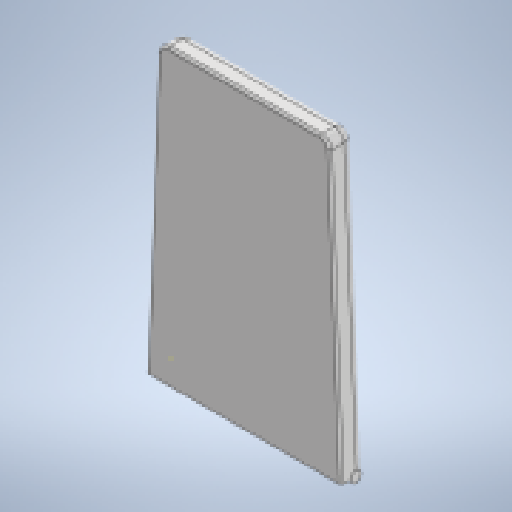
# Autodesk Inventor part: backrest wheelchair EG26
Saved by Autodesk Inventor 2023 (Build 270158000, 158)
## iProperties
Created: 2023-10-18
Part Number: backrest wheelchair EG26
Material: Generic
Document SubType Name: Modeling
Designer: user
Density: 1 g/cm^3
Appearance: Default
Author: user
Autodesk Inventor part; units mm, degrees
ref_plane "YZ Plane" through (0, 0, 0) normal (1, 0, 0) x (0, 1, 0)
ref_plane "XZ Plane" through (0, 0, 0) normal (0, 1, 0) x (-1, 0, 0)
ref_plane "XY Plane" through (0, 0, 0) normal (0, 0, 1) x (1, 0, 0)
sketch "Sketch1" plane through (0, 0, 0) normal (0, 0, 1) x (1, 0, 0)
  line L0 (0, 0) -> (25, 600)
  line L1 (25, 600) -> (375, 600)
  line L2 (375, 600) -> (400, 0)
  line L3 (400, 0) -> (0, 0)
  arc A0 (120.3096, 600) -> (279.6904, 600) centre (200, 673.1568) ccw
  line L4 (120.3096, 600) -> (25, 600)
  line L5 (25, 600) -> (0, 0)
  dimension "d0" = 600
  dimension "d1" = 25
  dimension "d2" = 350
  dimension "d3" = 400
  dimension "d4" = 175
  constraints: 12 end point, 2 point on circle, 2 point on line, 1 centre point, 1 collinear, 1 horizontal, 1 parallel
  measures "d0" vertical distance of L0.start L0.end
  measures "d1" horizontal distance of L0.start L0.end
  measures "d2" distance of L0.end L1.end
  measures "d3" distance of L2.end L0.start
  measures "d4" horizontal distance of L1.end A0.centre
extrude "Extrusion1" add sketch "Sketch1" along normal blind 50
fillet "Fillet1" radius 20 5 edges at (200, 600, 0) (387.5, 300, 0) (12.5, 300, 0) (25, 600, 25) (375, 600, 25)
fillet "Fillet2" radius 5 5 edges at (200, 600, 50) (30.3394, 594.4335, 50) (369.6606, 594.4335, 50) (387.8993, 290.4163, 50) (12.1007, 290.4163, 50)
sketch "Sketch2" plane through (0, 0, 0) normal (0, 0, 1) x (1, 0, 0)
  point P0 (0, 0)
sketch "Sketch3" plane through (0, 0, 0) normal (1, 0, 0) x (0, 1, 0)
  line L0 (0, 0) -> (0, 20) projected
  circle A0 centre (0, 20) radius 11.125
  dimension "d9" = 22.25
  constraints: 1 centre point
  measures "d9" diameter of A0
extrude "Extrusion2" add sketch "Sketch3" along normal blind 400
sketch "Sketch4" plane through (0, 0, 0) normal (0, 1, 0) x (-1, 0, 0)
  circle A0 centre (-325, 12.7) radius 11.5572
  circle A1 centre (-75, 12.7) radius 11.125
  line L0 (0, 31.125) -> (-400, 31.125) projected
  line L1 (-200, 31.125) -> (-350.8375, 31.125)
  point P0 (0, 0)
  dimension "d12" = 22.25
  dimension "d13" = 250
  dimension "d16" = 125
  constraints: 2 centre point, 2 end point, 2 midpoint, 1 point on line
  measures "d12" diameter of A1
  measures "d13" distance of A1.centre A0.centre
  measures "d16" horizontal distance of A0.centre point (-200, 31.125)
extrude "Extrusion3" add sketch "Sketch4" against normal blind 30
body "Solid1"
